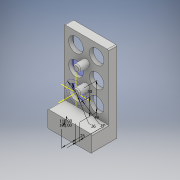
# Autodesk Inventor part: NespressoSpeedfiller-6X-long
Saved by Autodesk Inventor 2017 (Build 210142000, 142)
## iProperties
Created: 2018-08-27
Part Number: NespressoSpeedfiller-6X-long
Material: Generic
Document SubType Name: Modeling
Designer: 45027374
Density: 1 g/cm^3
Appearance: Default
Author: 45027374
Autodesk Inventor part; units mm, degrees
ref_plane "YZ Plane" through (0, 0, 0) normal (1, 0, 0) x (0, 1, 0)
ref_plane "XY Plane" through (0, 0, 0) normal (0, 0, 1) x (1, 0, 0)
sketch "Sketch1" plane through (0, 0, 0) normal (0, 1, 0) x (-1, 0, 0)
  line L0 (25.9, 0) -> (-25.9, 0) projected
  line L1 (0, -25.9) -> (0, 25.9) projected
  circle A0 centre (0, 0) radius 18.5 construction
  circle A1 centre (0, 0) radius 13 construction
  dimension "d0" = 37
  dimension "d1" = 26
  constraints: 2 centre point, 2 coincident
  measures "d0" diameter of A0
  measures "d1" diameter of A1
sketch "Sketch2" plane through (0, 0, 0) normal (0, 1, 0) x (-1, 0, 0)
  line L0 (36.8, 0) -> (-73.8, 0) projected
  line L1 (0, -44.2) -> (0, 118.2) projected
  line L2 (-58, 95) -> (-58, -21)
  line L3 (-58, -21) -> (21, -21)
  line L4 (21, -21) -> (21, 95)
  line L5 (-58, 95) -> (21, 95)
  circle A0 centre (-37, 0) radius 18.5 construction
  circle A1 centre (-37, 37) radius 18.5 construction
  circle A2 centre (-37, 74) radius 18.5 construction
  point P0 (0, 0)
  dimension "d29" = 21
  dimension "d30" = 95
  dimension "d109" = 58
  dimension "d110" = 21
  dimension "d111" = 37
  dimension "d112" = 37
  dimension "d113" = 37
  dimension "d114" = 37
  dimension "d115" = 37
  dimension "d116" = 37
  dimension "d117" = 37
  dimension "d118" = 37
  constraints: 8 end point, 3 centre point, 1 horizontal, 1 point on line
  measures "d29" distance between parallel lines of L0 L3
  measures "d30" distance between parallel lines of L5 L0
  measures "d109" distance between parallel lines of L2 L1
  measures "d110" distance between parallel lines of L1 L4
  measures "d111" diameter of A0
  measures "d112" diameter of A1
  measures "d113" diameter of A2
  measures "d114" distance from line of L1 A0.centre
  measures "d115" distance of A0.centre A1.centre
  measures "d116" distance from line of L1 A1.centre
  measures "d117" distance from line of L1 A2.centre
  measures "d118" distance of A1.centre A2.centre
extrude "Extrusion1" add sketch "Sketch2" along normal blind 7
sketch "Sketch6" plane through (0, 0, 0) normal (0, 1, 0) x (-1, 0, 0)
  line L0 (21, -21) -> (-58, -21) projected
  line L1 (21, 95) -> (21, -21) projected
  line L2 (-58, -21) -> (21, -21)
  line L3 (21, -21) -> (21, 95)
  line L4 (-58, 95) -> (-58, -21)
  line L5 (80.1765, 0) -> (-86.8627, 0) projected
  line L6 (0, -44.2) -> (0, 118.2) projected
  line L7 (21, 95) -> (-58, 95) projected
  line L8 (-53, 95) -> (-53, 0)
  line L9 (53, 0) -> (53, 95)
  line L10 (53, 95) -> (21, 95)
  line L11 (-58, 95) -> (-58, -21) projected
  line L12 (-58, 95) -> (-53, 95)
  arc A0 (37, -16) -> (53, 0) centre (37, 0) ccw
  arc A1 (-53, 0) -> (-37, -16) centre (-37, 0) ccw
  line L13 (37, -16) -> (-39.8141, -16)
  point P0 (0, 0)
  point P1 (-16, 0)
  dimension "d101" = 53
  dimension "d102" = 53
  dimension "d103" = 32
  dimension "d104" = 32
  constraints: 16 end point, 8 point on line, 4 point on circle, 3 perpendicular, 3 tangent, 2 centre point, 2 collinear, 2 parallel, 1 horizontal
  measures "d101" distance between parallel lines of L6 L8
  measures "d102" distance between parallel lines of L9 L6
  measures "d103" diameter of A1
  measures "d104" diameter of A0
extrude "Extrusion5" [suppressed]
sketch "Sketch4" plane through (0, 0, 0) normal (0, 0, 1) x (1, 0, 0)
  line L0 (-55.5, 0) -> (55.5, 0)
  line L1 (55.5, 0) -> (55.5, -2.5)
  line L2 (55.5, -2.5) -> (-55.5, -2.5)
  line L3 (-55.5, -2.5) -> (-55.5, 0)
  line L4 (-77.7, 0) -> (77.7, 0) projected
  line L5 (0, -3) -> (0, 0.5) projected
  point P0 (0, 0)
  dimension "d10" = 111
  dimension "d11" = 2.5
  constraints: 8 end point, 2 parallel, 1 collinear, 1 horizontal, 1 perpendicular, 1 other
  measures "d10" distance between parallel lines of L1 L3
  measures "d11" distance of L0.end L1.end
extrude "Extrusion6" [suppressed]
sketch "Sketch5" plane through (0, 0, 0) normal (0, 1, 0) x (-1, 0, 0)
  circle A0 centre (0, 0) radius 18.5 construction
  circle A1 centre (0, 0) radius 18.5 construction
  line L0 (77.7, 0) -> (-77.7, 0) projected
  line L1 (0, -28.9) -> (0, 26.4) projected
  line L2 (-55.5, -21) -> (55.5, -21)
  line L3 (55.5, -21) -> (55.5, -18.5)
  line L4 (55.5, -18.5) -> (-55.5, -18.5)
  line L5 (-55.5, -18.5) -> (-55.5, -21)
  dimension "d25" = 111
  dimension "d26" = 21
  constraints: 8 end point, 2 parallel, 1 centre point, 1 coincident, 1 concentric, 1 horizontal, 1 perpendicular, 1 tangent, 1 other
  measures "d25" distance of L2.start L2.end
  measures "d26" distance between parallel lines of L0 L2
extrude "Extrusion7" [suppressed]
sketch "Sketch7" plane through (0, 0, 0) normal (0, 0, 1) x (1, 0, 0)
  line L0 (-55.5, 0) -> (55.5, 0)
  line L1 (55.5, 0) -> (55.5, -2.5)
  line L2 (55.5, -2.5) -> (-55.5, -2.5)
  line L3 (-55.5, -2.5) -> (-55.5, 0)
  line L4 (58, 0) -> (-21, 0) projected
  line L5 (-79.2, 0) -> (86.7, 0) projected
  line L6 (0, -3) -> (0, 0.5) projected
  point P0 (-16, 0)
  point P1 (16, 0)
  point P2 (53, 0)
  point P3 (-53, 0)
  dimension "d53" = 2.5
  dimension "d54" = 55.5
  constraints: 8 end point, 2 parallel, 1 collinear, 1 horizontal, 1 perpendicular, 1 other
  measures "d53" distance of L0.end L1.end
  measures "d54" distance between parallel lines of L6 L1
extrude "Extrusion8" [suppressed]
sketch "Sketch8" plane through (0, 0, 0) normal (0, 1, 0) x (-1, 0, 0)
  circle A0 centre (0, 0) radius 13
  dimension "d34" = 26
  constraints: 1 centre point, 1 coincident
  measures "d34" diameter of A0
extrude "Extrusion9" cut sketch "Sketch8" along normal through all
pattern_linear "Rectangular Pattern1" count 3 spacing 37 along (0, 0, 1) count 2 spacing 37 along (1, 0, 0) of "Extrusion9" second direction both ways yes
sketch "Sketch9" plane through (0, 7, 0) normal (0, 1, 0) x (1, 0, 0)
  circle A0 centre (0, 0) radius 13
  circle A1 centre (0, 0) radius 15
  dimension "d40" = 26
  dimension "d41" = 30
  constraints: 2 centre point, 2 coincident
  measures "d40" diameter of A0
  measures "d41" diameter of A1
extrude "Extrusion10" [suppressed]
sketch "Sketch10" plane through (0, 5, 0) normal (0, 1, 0) x (1, 0, 0)
  arc A0 (16, 0) -> (-16, 0) centre (0, 0) ccw projected
  line L0 (1.5, -18) -> (-1.5, -18)
  line L1 (-29.4, 0) -> (29.4, 0) projected
  line L2 (0, 36.3) -> (0, -70.8) projected
  line L3 (1.5, -12) -> (-1.5, -12)
  line L4 (1.5, -12) -> (1.5, -18)
  line L5 (-1.5, -18) -> (-1.5, -12)
  dimension "d48" = 3
  dimension "d49" = 12
  dimension "d50" = 6
  constraints: 8 end point, 2 perpendicular, 1 horizontal, 1 parallel, 1 other
  measures "d48" distance between parallel lines of L4 L5
  measures "d49" distance between parallel lines of L1 L3
  measures "d50" distance between parallel lines of L0 L3
extrude "Extrusion11" [suppressed]
ref_plane "Work Plane1" through (0, 5, 0) normal (0, 1, 0) x (-1, 0, 0)
sketch "Sketch12" plane through (0, 5, 0) normal (0, 1, 0) x (-1, 0, 0)
  line L0 (21, -21) -> (-58, -21)
  line L1 (-58, -21) -> (-58, -51)
  line L2 (-58, -51) -> (21, -51)
  line L3 (21, -51) -> (21, -21)
  line L4 (43.8, 0) -> (-80.8, 0) projected
  line L5 (0, -64.9) -> (0, 32.4) projected
  point P0 (0, 0)
  dimension "d62" = 30
  dimension "d123" = 58
  dimension "d124" = 21
  dimension "d125" = 21
  constraints: 8 end point, 1 horizontal, 1 parallel, 1 perpendicular
  measures "d62" distance between parallel lines of L2 L0
  measures "d123" distance between parallel lines of L1 L5
  measures "d124" distance between parallel lines of L5 L3
  measures "d125" distance between parallel lines of L4 L0
extrude "Extrusion12" add sketch "Sketch12" against normal blind 34.5
sketch "Sketch13" plane through (0, 0, 0) normal (1, 0, 0) x (0, 1, 0)
  line L0 (-31.4, 0) -> (13.4, 0) projected
  line L1 (0, -62.5) -> (0, 32) projected
  line L2 (7, -19) -> (7, -49)
  line L3 (7, -49) -> (-25, -43.3575)
  line L4 (-25, -43.3575) -> (-25, -30.647)
  line L5 (7, -19) -> (-25, -30.647)
  point P0 (0, 0)
  dimension "d85" = 25
  dimension "d86" = 7
  dimension "d87" = 49
  dimension "d88" = 30
  dimension "d89" = 100
  dimension "d90" = 110
  constraints: 8 end point, 1 parallel, 1 vertical
  measures "d85" distance between parallel lines of L1 L4
  measures "d86" distance between parallel lines of L2 L1
  measures "d87" distance from line of L0 L2.end
  measures "d88" distance of L2.start L2.end
  measures "d89" angle of L4 L3
  measures "d90" angle of L5 L4
extrude "Extrusion14" cut sketch "Sketch13" against normal blind 19
sketch "Sketch14" plane through (0, 5, 0) normal (0, 1, 0) x (-1, 0, 0)
  line L0 (0, -80.2) -> (0, 124.2) projected
  line L1 (19, 93) -> (-56, 93)
  line L2 (-56, 93) -> (-56, -49)
  line L3 (-56, -49) -> (19, -49)
  line L4 (19, -49) -> (19, 93)
  line L5 (21, 95) -> (-58, 95)
  line L6 (-58, 95) -> (-58, -51)
  line L7 (-58, -51) -> (21, -51)
  line L8 (21, -51) -> (21, 95)
  line L9 (43.8, 0) -> (-80.8, 0) projected
  dimension "d91" = 51
  dimension "d92" = 95
  dimension "d95" = 93
  dimension "d96" = 49
  dimension "d119" = 58
  dimension "d120" = 21
  dimension "d121" = 56
  dimension "d122" = 19
  constraints: 16 end point, 2 horizontal, 2 parallel, 2 perpendicular
  measures "d91" distance between parallel lines of L7 L9
  measures "d92" distance between parallel lines of L5 L9
  measures "d95" distance between parallel lines of L1 L9
  measures "d96" distance between parallel lines of L9 L3
  measures "d119" distance between parallel lines of L0 L6
  measures "d120" distance between parallel lines of L0 L8
  measures "d121" distance between parallel lines of L0 L2
  measures "d122" distance between parallel lines of L0 L4
extrude "Extrusion15" add sketch "Sketch14" along normal blind 10 contours L7 L6 L9 L2 L3 L0 | L0 L3 L4 L9 L8 L7 | L6 L5 L0 L1 L2 L9 | L9 L4 L1 L0 L5 L8
fillet "Fillet3" radius 2 4 edges at (58, 7.5, 95) (58, -7.25, -51) (-21, -7.25, -51) (-21, 7.5, 95)
fillet "Fillet5" radius 2 2 edges at (58, -14.75, -21) (-21, -14.75, -21)
fillet "Fillet8" [suppressed]
extrude "Extrusion16" cut sketch "Sketch13" along normal blind 56
sketch "Sketch15" plane through (0, 0, 0) normal (0, 1, 0) x (-1, 0, 0)
  circle A0 centre (-18.5, 18.5) radius 5.875
  line L0 (27.075, 0) -> (-32.95, 0) projected
  line L1 (0, -34.475) -> (0, 77.35) projected
  circle A1 centre (-18.5, 55.5) radius 5.875
  point P0 (0, 0)
  dimension "d128" = 18.5
  dimension "d129" = 18.5
  dimension "d130" = 11.75
  dimension "d133" = 37
  constraints: 2 centre point, 1 vertical, 2 other
  measures "d128" distance from line of L0 A0.centre
  measures "d129" distance from line of L1 A0.centre
  measures "d130" diameter of A0
  measures "d133" distance of A0.centre A1.centre
extrude "Extrusion17" add sketch "Sketch15" against normal blind 18
fillet "Fillet9" radius 2 2 edges at (24.375, -18, 55.5) (24.375, -18, 18.5)
fillet "Fillet10" radius 4 2 edges at (18.5, -25, -43.3575) (18.5, -25, -30.647)
fillet "Fillet11" radius 2 1 edges at (18.5, 7, -19)
equation "\"d115\" = d114"
equation "\"d117\" = d116"
equation "\"d118\" = d115"
equation "\"d102\" = d101"
body "Solid1"
